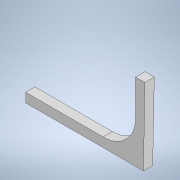
# Autodesk Inventor part: hOLD_2
Saved by Autodesk Inventor 2020 (Build 240168000, 168)
## iProperties
Created: 2021-02-07
Part Number: hOLD_2
Material: Generic
Document SubType Name: Modeling
Designer: moham
Density: 1 g/cm^3
Appearance: Default
Author: moham
Autodesk Inventor part; units mm, degrees
ref_plane "YZ Plane" through (0, 0, 0) normal (1, 0, 0) x (0, 1, 0)
ref_plane "XZ Plane" through (0, 0, 0) normal (0, 1, 0) x (-1, 0, 0)
ref_plane "XY Plane" through (0, 0, 0) normal (0, 0, 1) x (1, 0, 0)
sketch "Sketch1" plane through (0, 0, 0) normal (0, 0, 1) x (1, 0, 0)
  circle A0 centre (0, 0) radius 21
  line L0 (0, -21) -> (-50, -21)
  line L1 (-50, -21) -> (-50, -27)
  line L2 (-50, -27) -> (49, -27)
  line L3 (21, 0) -> (21, 23)
  line L4 (21, 23) -> (27, 23)
  line L5 (27, 23) -> (26, -27)
  dimension "d0" = 42
  dimension "d1" = 50
  dimension "d2" = 6
  dimension "d4" = 6
  dimension "d5" = 50
  constraints: 12 end point, 3 perpendicular, 2 point on circle, 1 centre point, 1 coincident, 1 horizontal, 1 point on line, 1 tangent, 1 vertical
  measures "d0" diameter of A0
  measures "d1" distance of L0.start L0.end
  measures "d2" distance of L0.end L1.end
  measures "d4" distance of L3.end L4.end
  measures "d5" vertical distance of L4.end L5.end
extrude "Extrusion1" add sketch "Sketch1" along normal blind 6 contours L3 L4 L5 L2 L1 L0 A0
body "Solid1"
